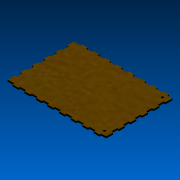
# Autodesk Inventor part: fond
Saved by Autodesk Inventor 2013 SP2 (Build 170200200, 200)
## iProperties
Created: 2015-09-15
Part Number: fond
Material: Generic
Document SubType Name: Modeling
Designer: jeanfrancois
Density: 1 g/cm^3
Author: jeanfrancois
Autodesk Inventor part; units mm, degrees
ref_plane "YZ Plane" through (0, 0, 0) normal (1, 0, 0) x (0, 1, 0)
ref_plane "XZ Plane" through (0, 0, 0) normal (0, 1, 0) x (-1, 0, 0)
ref_plane "XY Plane" through (0, 0, 0) normal (0, 0, 1) x (1, 0, 0)
sketch "Esquisse1" plane through (0, 0, 0) normal (0, 0, 1) x (1, 0, 0)
  line L0 (87.3006, 60.3174) -> (87.3006, 48.3174)
  line L1 (87.3006, 38.3174) -> (87.3006, 28.3174)
  line L2 (84.3006, 48.3174) -> (84.3006, 38.3174)
  line L3 (84.3006, 48.3174) -> (87.3006, 48.3174)
  line L4 (84.3006, 38.3174) -> (87.3006, 38.3174)
  line L5 (84.3006, 28.3174) -> (84.3006, 18.3174)
  line L6 (84.3006, 28.3174) -> (87.3006, 28.3174)
  line L7 (78.8006, 60.3174) -> (87.3006, 60.3174)
  line L8 (68.8006, 63.3174) -> (78.8006, 63.3174)
  line L9 (78.8006, 63.3174) -> (78.8006, 60.3174)
  line L10 (58.8006, 60.3174) -> (68.8006, 60.3174)
  line L11 (68.8006, 63.3174) -> (68.8006, 60.3174)
  line L12 (48.8006, 63.3174) -> (58.8006, 63.3174)
  line L13 (58.8006, 63.3174) -> (58.8006, 60.3174)
  line L14 (48.8006, 63.3174) -> (48.8006, 60.3174)
  line L15 (38.8006, 63.3174) -> (38.8006, 60.3174)
  line L16 (18.8006, 60.3174) -> (28.8006, 60.3174)
  line L17 (28.8006, 63.3174) -> (38.8006, 63.3174)
  line L18 (28.8006, 63.3174) -> (28.8006, 60.3174)
  line L19 (38.8006, 60.3174) -> (48.8006, 60.3174)
  line L20 (87.3006, 18.3174) -> (87.3006, 8.3174)
  line L21 (87.3006, -21.6826) -> (87.3006, -31.6826)
  line L22 (87.3006, -1.6826) -> (87.3006, -11.6826)
  line L23 (87.3006, -41.6826) -> (87.3006, -53.6826)
  line L24 (84.3006, -31.6826) -> (84.3006, -41.6826)
  line L25 (84.3006, -31.6826) -> (87.3006, -31.6826)
  line L26 (48.8006, -56.6826) -> (58.8006, -56.6826)
  line L27 (58.8006, -56.6826) -> (58.8006, -53.6826)
  line L28 (58.8006, -53.6826) -> (68.8006, -53.6826)
  line L29 (68.8006, -56.6826) -> (68.8006, -53.6826)
  line L30 (68.8006, -56.6826) -> (78.8006, -56.6826)
  line L31 (78.8006, -56.6826) -> (78.8006, -53.6826)
  line L32 (78.8006, -53.6826) -> (87.3006, -53.6826)
  line L33 (84.3006, -41.6826) -> (87.3006, -41.6826)
  line L34 (84.3006, -21.6826) -> (87.3006, -21.6826)
  line L35 (84.3006, -11.6826) -> (84.3006, -21.6826)
  line L36 (84.3006, -11.6826) -> (87.3006, -11.6826)
  line L37 (84.3006, 8.3174) -> (84.3006, -1.6826)
  line L38 (84.3006, 8.3174) -> (87.3006, 8.3174)
  line L39 (84.3006, 18.3174) -> (87.3006, 18.3174)
  line L40 (84.3006, -1.6826) -> (87.3006, -1.6826)
  line L41 (-1.1994, 60.3174) -> (8.8006, 60.3174)
  line L42 (-21.1994, 60.3174) -> (-11.1994, 60.3174)
  line L43 (-11.1994, 63.3174) -> (-11.1994, 60.3174)
  line L44 (-11.1994, 63.3174) -> (-1.1994, 63.3174)
  line L45 (-1.1994, 63.3174) -> (-1.1994, 60.3174)
  line L46 (8.8006, 63.3174) -> (8.8006, 60.3174)
  line L47 (18.8006, 63.3174) -> (18.8006, 60.3174)
  line L48 (8.8006, 63.3174) -> (18.8006, 63.3174)
  line L49 (38.8006, -56.6826) -> (38.8006, -53.6826)
  line L50 (38.8006, -53.6826) -> (48.8006, -53.6826)
  line L51 (28.8006, -56.6826) -> (28.8006, -53.6826)
  line L52 (28.8006, -56.6826) -> (38.8006, -56.6826)
  line L53 (18.8006, -53.6826) -> (28.8006, -53.6826)
  line L54 (18.8006, -56.6826) -> (18.8006, -53.6826)
  line L55 (8.8006, -56.6826) -> (8.8006, -53.6826)
  line L56 (8.8006, -56.6826) -> (18.8006, -56.6826)
  line L57 (-1.1994, -53.6826) -> (8.8006, -53.6826)
  line L58 (-1.1994, -56.6826) -> (-1.1994, -53.6826)
  line L59 (-11.1994, -56.6826) -> (-11.1994, -53.6826)
  line L60 (-11.1994, -56.6826) -> (-1.1994, -56.6826)
  line L61 (-21.1994, -53.6826) -> (-11.1994, -53.6826)
  line L62 (-21.1994, -56.6826) -> (-21.1994, -53.6826)
  line L63 (-31.1994, -56.6826) -> (-31.1994, -53.6826)
  line L64 (-31.1994, -56.6826) -> (-21.1994, -56.6826)
  line L65 (-41.1994, -53.6826) -> (-31.1994, -53.6826)
  line L66 (48.8006, -56.6826) -> (48.8006, -53.6826)
  line L67 (-82.6994, 28.3174) -> (-82.6994, 38.3174)
  line L68 (-82.6994, 48.3174) -> (-82.6994, 60.3174)
  line L69 (-79.6994, 38.3174) -> (-79.6994, 48.3174)
  line L70 (-79.6994, 48.3174) -> (-82.6994, 48.3174)
  line L71 (-79.6994, 38.3174) -> (-82.6994, 38.3174)
  line L72 (-79.6994, 18.3174) -> (-79.6994, 28.3174)
  line L73 (-79.6994, 28.3174) -> (-82.6994, 28.3174)
  line L74 (-41.1994, 60.3174) -> (-31.1994, 60.3174)
  line L75 (-21.1994, 63.3174) -> (-21.1994, 60.3174)
  line L76 (-31.1994, 63.3174) -> (-31.1994, 60.3174)
  line L77 (-41.1994, 63.3174) -> (-41.1994, 60.3174)
  line L78 (-51.1994, 63.3174) -> (-41.1994, 63.3174)
  line L79 (-51.1994, 63.3174) -> (-51.1994, 60.3174)
  line L80 (-61.1994, 60.3174) -> (-51.1994, 60.3174)
  line L81 (-61.1994, 63.3174) -> (-61.1994, 60.3174)
  line L82 (-71.1994, 63.3174) -> (-61.1994, 63.3174)
  line L83 (-71.1994, 63.3174) -> (-71.1994, 60.3174)
  line L84 (-82.6994, 60.3174) -> (-71.1994, 60.3174)
  line L85 (-31.1994, 63.3174) -> (-21.1994, 63.3174)
  line L86 (-82.6994, 8.3174) -> (-82.6994, 18.3174)
  line L87 (-82.6994, -53.6826) -> (-82.6994, -41.6826)
  line L88 (-82.6994, -31.6826) -> (-82.6994, -21.6826)
  line L89 (-82.6994, -11.6826) -> (-82.6994, -1.6826)
  line L90 (-79.6994, 18.3174) -> (-82.6994, 18.3174)
  line L91 (-79.6994, -41.6826) -> (-79.6994, -31.6826)
  line L92 (-79.6994, -31.6826) -> (-82.6994, -31.6826)
  line L93 (-79.6994, -41.6826) -> (-82.6994, -41.6826)
  line L94 (-79.6994, -21.6826) -> (-79.6994, -11.6826)
  line L95 (-79.6994, -11.6826) -> (-82.6994, -11.6826)
  line L96 (-79.6994, -1.6826) -> (-79.6994, 8.3174)
  line L97 (-79.6994, -21.6826) -> (-82.6994, -21.6826)
  line L98 (-79.6994, 8.3174) -> (-82.6994, 8.3174)
  line L99 (-79.6994, -1.6826) -> (-82.6994, -1.6826)
  line L100 (-41.1994, -56.6826) -> (-41.1994, -53.6826)
  line L101 (-51.1994, -56.6826) -> (-41.1994, -56.6826)
  line L102 (-51.1994, -56.6826) -> (-51.1994, -53.6826)
  line L103 (-61.1994, -53.6826) -> (-51.1994, -53.6826)
  line L104 (-71.1994, -56.6826) -> (-61.1994, -56.6826)
  line L105 (-71.1994, -56.6826) -> (-71.1994, -53.6826)
  line L106 (-82.6994, -53.6826) -> (-71.1994, -53.6826)
  line L107 (-61.1994, -56.6826) -> (-61.1994, -53.6826)
  point P0 (0, 0)
  constraints: 216 end point
extrude "Extrusion1" add sketch "Esquisse1" along normal blind 3
hole "Perçage1" at (77.3006, 53.3174, 3) direction (0, 0, -1) diameter 4 end through all
hole "Perçage2" at (77.3006, -46.6826, 3) direction (0, 0, -1) diameter 4 end through all
